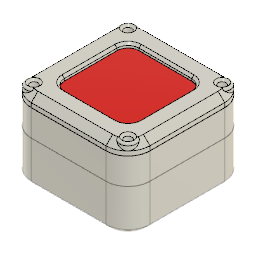
EmergencyButton (Autodesk Fusion 360 design; units mm, degrees)
Autodesk Fusion 360 part; units mm, degrees
note: some values were not read from the file. Chosen so that the rebuilt part matches the saved one: which face or edge a step refers to. Set by a fixed rule: which sketch regions a step uses.
sketch "Sketch1" plane through (0, 0, 0) normal (0, 0, 1) x (1, 0, 0) in component "Lower"
  line L0 (27, 27) -> (-27, 27)
  line L1 (-27, 27) -> (-27, -27)
  line L2 (-27, -27) -> (27, -27)
  line L3 (27, -27) -> (27, 27)
  line L4 (27, 27) -> (-27, -27) construction
  line L5 (-27, 27) -> (27, -27) construction
  dimension "d1" = 54
  dimension "d2" = 54
extrude "Extrude1" add sketch "Sketch1" along normal blind 19 makes body 1 in component "Lower"
fillet "Fillet1" radius 10 4 edges at (-27, -27, 9.5) (27, -27, 9.5) (27, 27, 9.5) (-27, 27, 9.5) on bodies 1 in component "Lower"
chamfer "Chamfer1" distance 2 angle 45 8 edges at (0, 27, 0) (-24.0711, 24.0711, 0) (-27, 0, 0) (-24.0711, -24.0711, 0) (0, -27, 0) (24.0711, -24.0711, 0) (27, 0, 0) (24.0711, 24.0711, 0) on bodies 1 in component "Lower"
shell "Shell1" thickness 2 removed faces 1 at (5.6667, -9, 19) on bodies 1 in component "Lower"
sketch "Sketch1 (2)" plane through (0, 0, 19) normal (0, 0, 1) x (-1, 0, 0) in component "Middle"
  arc A0 (-17, 25) -> (-25, 17) centre (-17, 17) ccw
  line L0 (-17, 25) -> (17, 25)
  arc A1 (25, 17) -> (17, 25) centre (17, 17) ccw
  line L1 (25, 17) -> (25, -17)
  arc A2 (17, -25) -> (25, -17) centre (17, -17) ccw
  line L2 (17, -25) -> (-17, -25)
  arc A3 (-25, -17) -> (-17, -25) centre (-17, -17) ccw
  line L3 (-25, -17) -> (-25, 17)
  arc A4 (17, -27) -> (27, -17) centre (17, -17) ccw
  line L4 (27, -17) -> (27, 17)
  arc A5 (27, 17) -> (17, 27) centre (17, 17) ccw
  line L5 (17, 27) -> (-17, 27)
  arc A6 (-17, 27) -> (-27, 17) centre (-17, 17) ccw
  line L6 (-27, 17) -> (-27, -17)
  arc A7 (-27, -17) -> (-17, -27) centre (-17, -17) ccw
  line L7 (-17, -27) -> (17, -27)
extrude "Extrude1'" add sketch "Sketch1 (2)" along normal blind 2 separate body contours A0 L0 A1 L1 A2 L2 A3 L3 | A4 L4 A5 L5 A6 L6 A7 L7 makes body 2 in component "Middle"
sketch "Sketch3" plane through (0, 0, 21) normal (0, 0, 1) x (-1, 0, 0) in component "Middle"
  line L0 (-17, -27) -> (17, -27)
  arc A0 (17, -27) -> (27, -17) centre (17, -17) ccw
  line L1 (27, -17) -> (27, 17)
  arc A1 (27, 17) -> (17, 27) centre (17, 17) ccw
  line L2 (17, 27) -> (-17, 27)
  arc A2 (-17, 27) -> (-27, 17) centre (-17, 17) ccw
  line L3 (-27, 17) -> (-27, -17)
  arc A3 (-27, -17) -> (-17, -27) centre (-17, -17) ccw
  line L4 (17, 19) -> (-17, 19)
  arc A4 (-17, 19) -> (-19, 17) centre (-17, 17) ccw
  line L5 (-19, 17) -> (-19, -17)
  arc A5 (-19, -17) -> (-17, -19) centre (-17, -17) ccw
  line L6 (-17, -19) -> (17, -19)
  arc A6 (17, -19) -> (19, -17) centre (17, -17) ccw
  line L7 (19, -17) -> (19, 17)
  arc A7 (19, 17) -> (17, 19) centre (17, 17) ccw
  dimension "d16" = 8
  measures "d16" distance of L2
extrude "Extrude2" add sketch "Sketch3" along normal blind 10 bodies 2 in component "Middle"
ref_plane "WorkPlane1" through (0, 0, 26.6) normal (0, 0, 1) x (-1, 0, 0) in component "TriggerButton"
sketch "Sketch1 (3)" plane through (0, 0, 26.6) normal (0, 0, 1) x (1, 0, 0) in component "TriggerButton"
  line L0 (-17, 19) -> (17, 19)
  arc A0 (19, 17) -> (17, 19) centre (17, 17) ccw
  line L1 (19, 17) -> (19, -17)
  arc A1 (17, -19) -> (19, -17) centre (17, -17) ccw
  line L2 (17, -19) -> (-17, -19)
  line L3 (-19, -17) -> (-19, 17)
  arc A2 (-19, -17) -> (-17, -19) centre (-17, -17) ccw
  arc A3 (-17, 19) -> (-19, 17) centre (-17, 17) ccw
  arc A4 (18.7, 17) -> (17, 18.7) centre (17, 17) ccw
  line L4 (-17, 18.7) -> (17, 18.7)
  arc A5 (-17, 18.7) -> (-18.7, 17) centre (-17, 17) ccw
  line L5 (-18.7, -17) -> (-18.7, 17)
  arc A6 (-18.7, -17) -> (-17, -18.7) centre (-17, -17) ccw
  line L6 (17, -18.7) -> (-17, -18.7)
  arc A7 (17, -18.7) -> (18.7, -17) centre (17, -17) ccw
  line L7 (18.7, 17) -> (18.7, -17)
  dimension "d21" = 0.3
extrude "Extrude1''" add sketch "Sketch1 (3)" along normal blind 4.4 separate body contours A4 L4 A5 L5 A6 L6 A7 L7 makes body 3 in component "TriggerButton"
sketch "Sketch2" plane through (0, 0, 31) normal (0, 0, 1) x (-1, 0, 0) in component "TriggerButton"
  arc A0 (17, -18.7) -> (18.7, -17) centre (17, -17) ccw
  line L0 (18.7, -17) -> (18.7, 17)
  arc A1 (18.7, 17) -> (17, 18.7) centre (17, 17) ccw
  line L1 (17, 18.7) -> (-17, 18.7)
  arc A2 (-17, 18.7) -> (-18.7, 17) centre (-17, 17) ccw
  line L2 (-18.7, 17) -> (-18.7, -17)
  arc A3 (-18.7, -17) -> (-17, -18.7) centre (-17, -17) ccw
  line L3 (-17, -18.7) -> (17, -18.7)
extrude "Extrude2'" add sketch "Sketch2" along normal blind 3 bodies 3 in component "TriggerButton"
sketch "Sketch1 (4)" plane through (0, 0, 31) normal (0, 0, 1) x (-1, 0, 0) in component "Upper"
  arc A0 (19, 17) -> (17, 19) centre (17, 17) ccw
  line L0 (19, 17) -> (19, -17)
  arc A1 (17, -19) -> (19, -17) centre (17, -17) ccw
  line L1 (17, -19) -> (-17, -19)
  arc A2 (-19, -17) -> (-17, -19) centre (-17, -17) ccw
  line L2 (-19, -17) -> (-19, 17)
  arc A3 (-17, 19) -> (-19, 17) centre (-17, 17) ccw
  line L3 (-17, 19) -> (17, 19)
  arc A4 (-27, -17) -> (-17, -27) centre (-17, -17) ccw
  line L4 (-17, -27) -> (17, -27)
  arc A5 (17, -27) -> (27, -17) centre (17, -17) ccw
  line L5 (27, -17) -> (27, 17)
  arc A6 (27, 17) -> (17, 27) centre (17, 17) ccw
  line L6 (17, 27) -> (-17, 27)
  arc A7 (-17, 27) -> (-27, 17) centre (-17, 17) ccw
  line L7 (-27, 17) -> (-27, -17)
extrude "Extrude1'''" add sketch "Sketch1 (4)" along normal blind 5 separate body contours A0 L0 A1 L1 A2 L2 A3 L3 | A4 L4 A5 L5 A6 L6 A7 L7 makes body 4 in component "Upper"
sketch "Sketch4" plane through (0, 0, 31) normal (0, 0, -1) x (1, 0, 0) in component "Upper"
  line L0 (27, -17) -> (27, 17)
  arc A0 (27, 17) -> (17, 27) centre (17, 17) ccw
  line L1 (17, 27) -> (-17, 27)
  arc A1 (-17, 27) -> (-27, 17) centre (-17, 17) ccw
  line L2 (-27, 17) -> (-27, -17)
  arc A2 (-27, -17) -> (-17, -27) centre (-17, -17) ccw
  line L3 (-17, -27) -> (17, -27)
  arc A3 (17, -27) -> (27, -17) centre (17, -17) ccw
  arc A4 (-18.7, -17) -> (-17, -18.7) centre (-17, -17) ccw
  line L4 (-17, -18.7) -> (17, -18.7)
  arc A5 (17, -18.7) -> (18.7, -17) centre (17, -17) ccw
  line L5 (18.7, -17) -> (18.7, 17)
  arc A6 (18.7, 17) -> (17, 18.7) centre (17, 17) ccw
  line L6 (17, 18.7) -> (-17, 18.7)
  arc A7 (-17, 18.7) -> (-18.7, 17) centre (-17, 17) ccw
  line L7 (-18.7, 17) -> (-18.7, -17)
  line L8 (-19, 17) -> (-19, -17)
  arc A8 (-19, -17) -> (-17, -19) centre (-17, -17) ccw
  line L9 (-17, -19) -> (17, -19)
  arc A9 (17, -19) -> (19, -17) centre (17, -17) ccw
  line L10 (19, -17) -> (19, 17)
  arc A10 (19, 17) -> (17, 19) centre (17, 17) ccw
  line L11 (17, 19) -> (-17, 19)
  arc A11 (-17, 19) -> (-19, 17) centre (-17, 17) ccw
  dimension "d72" = 0.3
  measures "d72" distance of L7
extrude "Extrude5" cut sketch "Sketch4" against normal blind 3 contours A4 L4 A5 L5 A6 L6 A7 L7 | L8 A8 L9 A9 L10 A10 L11 A11 bodies 4 in component "Upper"
sketch "Sketch5" plane through (0, 0, 34) normal (0, 0, -1) x (1, 0, 0) in component "Upper"
  arc A0 (-17, 19) -> (-19, 17) centre (-17, 17) ccw
  line L0 (-19, 17) -> (-19, -17)
  arc A1 (-19, -17) -> (-17, -19) centre (-17, -17) ccw
  line L1 (-17, -19) -> (17, -19)
  arc A2 (17, -19) -> (19, -17) centre (17, -17) ccw
  line L2 (19, -17) -> (19, 17)
  arc A3 (19, 17) -> (17, 19) centre (17, 17) ccw
  line L3 (17, 19) -> (-17, 19)
  line L4 (-17, 12) -> (-17, -12)
  line L5 (-12, -17) -> (12, -17)
  line L6 (17, -12) -> (17, 12)
  line L7 (12, 17) -> (-12, 17)
  arc A4 (-12, 17) -> (-17, 12) centre (-12, 12) ccw
  arc A5 (17, 12) -> (12, 17) centre (12, 12) ccw
  arc A6 (12, -17) -> (17, -12) centre (12, -12) ccw
  arc A7 (-17, -12) -> (-12, -17) centre (-12, -12) ccw
  dimension "d79" = 5
  measures "d79" radius of A4
extrude "Extrude2''" cut sketch "Sketch5" against normal up to surface (2 mm away) contours L4 L5 L6 L7 A4 A5 A6 A7 bodies 4 in component "Upper"
chamfer "Chamfer1'" distance 3 angle 45 8 edges at (0, -27, 36) (24.0711, -24.0711, 36) (27, 0, 36) (24.0711, 24.0711, 36) (0, 27, 36) (-24.0711, 24.0711, 36) (-27, 0, 36) (-24.0711, -24.0711, 36) on bodies 4 in component "Upper"
sketch "Sketch1 (1)" plane through (0, 0, 19) normal (0, 0, 1) x (-1, 0, 0) in component "Lower"
  arc A0 (-17, 25) -> (-25, 17) centre (-17, 17) ccw
  line L0 (-17, 25) -> (17, 25)
  arc A1 (25, 17) -> (17, 25) centre (17, 17) ccw
  line L1 (25, 17) -> (25, -17)
  arc A2 (17, -25) -> (25, -17) centre (17, -17) ccw
  line L2 (17, -25) -> (-17, -25)
  arc A3 (-25, -17) -> (-17, -25) centre (-17, -17) ccw
  line L3 (-25, -17) -> (-25, 17)
  arc A4 (17, -27) -> (27, -17) centre (17, -17) ccw
  line L4 (27, -17) -> (27, 17)
  arc A5 (27, 17) -> (17, 27) centre (17, 17) ccw
  line L5 (17, 27) -> (-17, 27)
  arc A6 (-17, 27) -> (-27, 17) centre (-17, 17) ccw
  line L6 (-27, 17) -> (-27, -17)
  arc A7 (-27, -17) -> (-17, -27) centre (-17, -17) ccw
  line L7 (-17, -27) -> (17, -27)
  circle A8 centre (21.4194, 21.4194) radius 3.75
  line L8 (22.6569, 22.6569) -> (24.0711, 24.0711) construction
  line L9 (22.6569, 22.6569) -> (21.4194, 21.4194) construction
  circle A9 centre (21.4194, 21.4194) radius 1.55
  dimension "d34" = 7.5
  dimension "d40" = 3.1
  measures "d34" diameter of A8
  measures "d40" diameter of A9
extrude "Extrude1''''" add sketch "Sketch1 (1)" against normal up to surface (19 mm away) contours A1 A8 | A9 picked at (23.689, 19.947) bodies 1 in component "Lower"
extrude "Extrude2'''" cut sketch "Sketch1 (1)" against normal up to surface (19 mm away) contours A9 bodies 1 in component "Lower"
ref_plane "WorkPlane1" through (0, 0, 10.9142) normal (-1, 0, 0) x (0, -1, 0) in component "Lower"
mirror "Mirror1" about plane through (0, 0, 10.9142) normal (-1, 0, 0) of "Extrude1''''", "Extrude2'''" in component "Lower"
ref_plane "WorkPlane2" through (0, 0, 10.9142) normal (0, 1, 0) x (-1, 0, 0) in component "Lower"
mirror "Mirror2" about plane through (0, 0, 10.9142) normal (0, 1, 0) of "Extrude1''''", "Extrude2'''", "Mirror1" in component "Lower"
sketch "Sketch4 (2)" plane through (0, 0, 31) normal (0, 0, 1) x (-1, 0, 0) in component "Middle"
  arc A0 (19, 17) -> (17, 19) centre (17, 17) ccw
  line L0 (19, 17) -> (19, -17)
  arc A1 (17, -19) -> (19, -17) centre (17, -17) ccw
  line L1 (17, -19) -> (-17, -19)
  arc A2 (-19, -17) -> (-17, -19) centre (-17, -17) ccw
  line L2 (-19, -17) -> (-19, 17)
  arc A3 (-17, 19) -> (-19, 17) centre (-17, 17) ccw
  line L3 (-17, 19) -> (17, 19)
  arc A4 (-27, -17) -> (-17, -27) centre (-17, -17) ccw
  line L4 (-17, -27) -> (17, -27)
  arc A5 (17, -27) -> (27, -17) centre (17, -17) ccw
  line L5 (27, -17) -> (27, 17)
  arc A6 (27, 17) -> (17, 27) centre (17, 17) ccw
  line L6 (17, 27) -> (-17, 27)
  arc A7 (-17, 27) -> (-27, 17) centre (-17, 17) ccw
  line L7 (-27, 17) -> (-27, -17)
  circle A8 centre (21.4194, 21.4194) radius 3.75
  circle A9 centre (21.4194, 21.4194) radius 1.75
  dimension "d43" = 3.5
  measures "d43" diameter of A9
extrude "Extrude3" cut sketch "Sketch4 (2)" against normal up to surface (12 mm away) contours A9 bodies 2 in component "Middle"
ref_plane "WorkPlane1" through (0, 0, 26) normal (-1, 0, 0) x (0, -1, 0) in component "Middle"
ref_plane "WorkPlane2" through (0, 0, 26) normal (0, -1, 0) x (1, 0, 0) in component "Middle"
mirror "Mirror1'" about plane through (0, 0, 26) normal (-1, 0, 0) of "Extrude3" in component "Middle"
mirror "Mirror2'" about plane through (0, 0, 26) normal (0, -1, 0) of "Extrude3", "Mirror1'" in component "Middle"
sketch "Sketch5 (2)" plane through (0, 0, 21) normal (0, 0, 1) x (-1, 0, 0) in component "Middle"
  line L0 (17, 19) -> (-17, 19)
  arc A0 (-17, 19) -> (-19, 17) centre (-17, 17) ccw
  line L1 (-19, 17) -> (-19, -17)
  arc A1 (-19, -17) -> (-17, -19) centre (-17, -17) ccw
  line L2 (-17, -19) -> (17, -19)
  arc A2 (17, -19) -> (19, -17) centre (17, -17) ccw
  line L3 (19, -17) -> (19, 17)
  arc A3 (19, 17) -> (17, 19) centre (17, 17) ccw
  line L4 (19, -17) -> (-19, -17)
  line L5 (17, -19) -> (17, 19)
  line L6 (-19, 17) -> (19, 17)
  line L7 (-17, 19) -> (-17, -19)
extrude "Extrude4" add sketch "Sketch5 (2)" along normal blind 4.4 contours L0 L5 L6 L7 | A3 L5 L6 | A0 L6 L7 | L3 L4 L5 L6 | L1 L4 L6 L7 | A2 L4 L5 | L2 L4 L5 L7 | A1 L4 L7 bodies 2 in component "Middle"
sketch "Sketch6" plane through (0, 0, 21) normal (0, 0, 1) x (-1, 0, 0) in component "Middle"
  line L0 (17, 17) -> (-17, 17)
  line L1 (-17, 17) -> (-17, -17)
  line L2 (-17, -17) -> (17, -17)
  line L3 (17, -17) -> (17, 17)
  line L4 (-3.4, -2.1) -> (3.4, -2.1)
  line L5 (3.4, -2.1) -> (3.4, 2.1)
  line L6 (3.4, 2.1) -> (-3.4, 2.1)
  line L7 (-3.4, 2.1) -> (-3.4, -2.1)
  line L8 (-3.4, -2.1) -> (3.4, 2.1) construction
  line L9 (3.4, -2.1) -> (-3.4, 2.1) construction
  circle A0 centre (3.4, -2.1) radius 1
  circle A1 centre (-3.4, -2.1) radius 1
  circle A2 centre (-3.4, 2.1) radius 1
  circle A3 centre (3.4, 2.1) radius 1
  dimension "d53" = 4.2
  dimension "d54" = 6.8
  dimension "d56" = 2
  dimension "d57" = 2
  dimension "d58" = 2
  dimension "d59" = 2
  measures "d56" diameter of A0
  measures "d57" diameter of A1
  measures "d58" diameter of A2
  measures "d59" diameter of A3
extrude "Extrude5'" cut sketch "Sketch6" against normal up to surface (2 mm away) contours L4 L7 A1 | L4 L7 A1 | L4 L5 A0 | L4 L5 A0 | L6 L7 A2 | L6 L7 A2 | L5 L6 A3 | L5 L6 A3 bodies 2 in component "Middle"
sketch "Sketch3 (2)" plane through (0, 0, 36) normal (0, 0, 1) x (-1, 0, 0) in component "Upper"
  line L0 (17, 24) -> (-17, 24)
  arc A0 (-17, 24) -> (-24, 17) centre (-17, 17) ccw
  line L1 (-24, 17) -> (-24, -17)
  arc A1 (-24, -17) -> (-17, -24) centre (-17, -17) ccw
  line L2 (-17, -24) -> (17, -24)
  arc A2 (17, -24) -> (24, -17) centre (17, -17) ccw
  line L3 (24, -17) -> (24, 17)
  arc A3 (24, 17) -> (17, 24) centre (17, 17) ccw
  circle A4 centre (21.4194, 21.4194) radius 1.75
  circle A5 centre (21.4194, 21.4194) radius 3.75
  line L4 (-12, 17) -> (12, 17)
  arc A6 (17, 12) -> (12, 17) centre (12, 12) ccw
  line L5 (17, 12) -> (17, -12)
  arc A7 (12, -17) -> (17, -12) centre (12, -12) ccw
  line L6 (12, -17) -> (-12, -17)
  arc A8 (-17, -12) -> (-12, -17) centre (-12, -12) ccw
  line L7 (-17, -12) -> (-17, 12)
  arc A9 (-12, 17) -> (-17, 12) centre (-12, 12) ccw
  dimension "d62" = 2
extrude "Extrude3'" add sketch "Sketch3 (2)" against normal up to surface (5 mm away) contours A3 A4 A5 | A3 A4 A5 bodies 4 in component "Upper"
extrude "Extrude4'" cut sketch "Sketch3 (2)" against normal up to surface (5 mm away) contours A3 A4 | A3 A4 bodies 4 in component "Upper"
fillet "Fillet1'" radius 1 1 edges at (-24.0711, -24.0711, 36) on bodies 4 in component "Upper"
ref_plane "WorkPlane1" through (0, 0, 35) normal (-1, 0, 0) x (0, -1, 0) in component "Upper"
ref_plane "WorkPlane2" through (0, 0, 35) normal (0, 1, 0) x (-1, 0, 0) in component "Upper"
mirror "Mirror1''" about plane through (0, 0, 35) normal (0, 1, 0) of "Extrude3'", "Extrude4'", "Fillet1'" in component "Upper"
mirror "Mirror2''" about plane through (0, 0, 35) normal (-1, 0, 0) of "Extrude3'", "Extrude4'", "Fillet1'", "Mirror1''" in component "Upper"
chamfer "Chamfer4" distance 1 angle 45 4 edges at (-19.7878, 20.7866, 36) (-19.7878, -22.0522, 36) (19.7878, -20.7866, 36) (19.7878, 22.0522, 36) on bodies 4 in component "Upper"
chamfer "Chamfer6" distance 1 angle 45 8 edges at (0, 17, 36) (15.5355, 15.5355, 36) (17, 0, 36) (15.5355, -15.5355, 36) (0, -17, 36) (-15.5355, -15.5355, 36) (-17, 0, 36) (-15.5355, 15.5355, 36) on bodies 4 in component "Upper"
component "Lower" placed x (1, 0, 0) y (0, 1, 0) z (0, 0, 1) at (0, 0, 0)
component "Middle" placed x (1, 0, 0) y (0, 1, 0) z (0, 0, 1) at (0, 0, 0)
component "TriggerButton" placed x (1, 0, 0) y (0, 1, 0) z (0, 0, 1) at (0, 0, 0)
component "Upper" placed x (1, 0, 0) y (0, 1, 0) z (0, 0, 1) at (0, 0, 0)
equation "d1 = ButtonWidth + 2 * WallThickness"
equation "d2 = ButtonHeight + 2 * WallThickness"
equation "WallThickness = 2 mm"
equation "ButtonWidth = 50 mm"
equation "ButtonHeight = 50 mm"
equation "LowerHeight = 17 mm"
equation "d7 = LowerHeight + WallThickness"
equation "d9 = WallThickness"
equation "d12 = WallThickness"
equation "PushButtonHeight = 5 mm"
equation "TriggerButtonLowerHeight = 5 mm"
equation "d17 = PushButtonHeight + TriggerButtonLowerHeight"
equation "tolerance = 0.3 mm"
equation "d20 = 2 * tolerance + PushButtonHeight"
equation "d21 = tolerance"
equation "d22 = TriggerButtonLowerHeight - ( 2 * tolerance )"
equation "TriggerButtonUpperHeight = 3 mm"
equation "d25 = TriggerButtonUpperHeight"
equation "d28 = TriggerButtonUpperHeight + WallThickness"
equation "d34 = 3.5 mm + 2 * WallThickness"
equation "PushWayPushButton = 0.3 mm"
equation "d49 = PushButtonHeight - PushWayPushButton - 0.3 mm"
equation "PinLegWidth = 4.2 mm"
equation "PinLegHeight = 6.8 mm"
equation "d53 = PinLegWidth"
equation "d54 = PinLegHeight"
equation "PinLegHoleDiameter = 2 mm"
equation "d56 = PinLegHoleDiameter"
equation "d57 = PinLegHoleDiameter"
equation "d58 = PinLegHoleDiameter"
equation "d59 = PinLegHoleDiameter"
equation "d62 = WallThickness"
equation "d72 = tolerance"
equation "d73 = -( TriggerButtonUpperHeight )"
